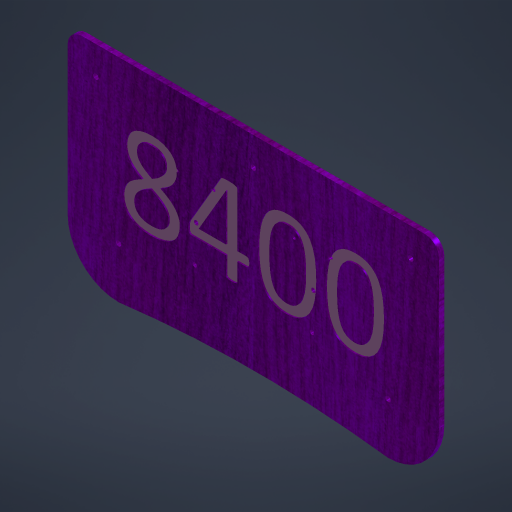
# Autodesk Inventor part: FTC Outside Panels
Saved by Autodesk Inventor 2024.2 (Build 282272000, 272)
## iProperties
Created: 2022-09-22
Part Number: FTC Outside Panels
Material: Wood (Oak)
Document SubType Name: Modeling
Designer: Jason
Density: 0.76 g/cm^3
Appearance: Birch - Natural Polished
Mass: 371.39 g
Surface Area: 1832.51 cm^2
Volume: 488.671 cm^3
Author: Allan
Autodesk Inventor part; units mm, degrees
ref_plane "YZ Plane" through (0, 0, 0) normal (1, 0, 0) x (0, 1, 0)
ref_plane "XZ Plane" through (0, 0, 0) normal (0, 1, 0) x (-1, 0, 0)
ref_plane "XY Plane" through (0, 0, 0) normal (0, 0, 1) x (1, 0, 0)
sketch "Sketch1" plane through (0, 0, 0) normal (0, 0, 1) x (1, 0, 0)
  line L0 (0, 0) -> (333.375, 0)
  line L1 (333.375, 0) -> (333.375, 177.8)
  line L2 (320.675, 190.5) -> (12.7, 190.5)
  line L3 (0, 177.8) -> (0, 0)
  circle A0 centre (45.72, 45.72) radius 45.72
  circle A1 centre (287.655, 45.72) radius 45.72
  line L4 (166.6875, 0) -> (166.6875, 7.62)
  arc A2 (287.655, 0) -> (45.72, 0) centre (166.6875, -956.3695) ccw
  arc A3 (12.7, 190.5) -> (0, 177.8) centre (12.7, 177.8) ccw
  arc A4 (333.375, 177.8) -> (320.675, 190.5) centre (320.675, 177.8) ccw
  circle A5 centre (45.72, 45.72) radius 2.413
  circle A6 centre (287.655, 45.72) radius 2.413
  circle A7 centre (25.4, 165.1) radius 2.413
  circle A8 centre (307.975, 165.1) radius 2.413
  line L5 (25.4, 165.1) -> (307.975, 165.1)
  circle A9 centre (166.6875, 165.1) radius 2.413
  ellipse E0 centre (219.2782, 63.3371) end of major axis (219.2708, 65.3371) minor radius 2
  line L6 (219.2782, 45.72) -> (219.2782, 63.3371)
  ellipse E1 centre (114.0968, 63.3371) end of major axis (114.0894, 65.3371) minor radius 2
  line L7 (114.0968, 45.72) -> (114.0968, 63.3371)
  circle A10 centre (219.3091, 79.3382) radius 4.699
  circle A11 centre (114.1277, 79.3382) radius 4.699
  line L8 (219.2782, 95.3392) -> (219.2782, 63.3371)
  line L9 (114.0968, 95.337) -> (114.0968, 63.3371)
  line L10 (45.72, 45.72) -> (114.0968, 45.72)
  line L11 (287.655, 45.72) -> (219.2782, 45.72)
  ellipse E2 centre (235.2526, 128.7087) end of major axis (235.2552, 127.3562) minor radius 1.3525
  ellipse E3 centre (203.2527, 128.6472) end of major axis (203.2553, 127.2947) minor radius 1.3525
  ellipse E4 centre (219.2782, 95.3392) end of major axis (219.2743, 97.3392) minor radius 2
  ellipse E5 centre (219.2782, 95.3392) end of major axis (219.2743, 97.3392) minor radius 2
  ellipse E6 centre (130.0712, 128.7066) end of major axis (130.0738, 127.354) minor radius 1.3525
  ellipse E7 centre (98.0713, 128.6451) end of major axis (98.0739, 127.2925) minor radius 1.3525
  ellipse E8 centre (114.0968, 95.337) end of major axis (114.0929, 97.337) minor radius 2
  ellipse E9 centre (114.0968, 95.337) end of major axis (114.0929, 97.337) minor radius 2
  point P0 (333.375, 190.5)
  point P1 (0, 190.5)
  point P2 (0, 45.72)
  point P3 (333.375, 45.72)
  dimension "d79" = 91.44
  dimension "d80" = 91.44
  dimension "d77" = 333.375
  dimension "d78" = 190.5
  dimension "d81" = 7.62
  dimension "d82" = 12.7
  dimension "d84" = 4.826
  dimension "d85" = 4.826
  dimension "d86" = 4.826
  dimension "d87" = 25.4
  dimension "d88" = 25.4
  dimension "d90" = 4.826
  dimension "d91" = 25.4
  dimension "d92" = 25.4
  dimension "d94" = 4.826
  dimension "d95" = 17.6171
  dimension "d97" = 17.6171
  dimension "d98" = 9.398
  dimension "d99" = 9.398
  dimension "d103" = 68.3768
  dimension "d104" = 68.3768
  constraints: 24 end point, 14 centre point, 7 point on circle, 6 point on line, 6 vertical, 5 horizontal, 4 tangent, 2 coincident, 2 midpoint, 2 parallel, 1 equal radius, 1 perpendicular, 18 other
  measures "d77" distance of point (0, 190.5) point (333.375, 190.5)
  measures "d78" distance of point (333.375, 190.5) L0.end
  measures "d81" distance of L4.start L4.end
  measures "d82" radius of A3
  measures "d84" diameter of A5
  measures "d85" diameter of A6
  measures "d86" diameter of A7
  measures "d87" distance from line of L2 L5.start
  measures "d88" distance from line of L3 L5.start
  measures "d90" diameter of A8
  measures "d91" distance from line of L1 L5.end
  measures "d92" distance from line of L2 L5.end
  measures "d94" diameter of A9
  measures "d95" distance of L6.start L6.end
  measures "d97" distance of L7.start L7.end
  measures "d98" diameter of A10
  measures "d99" diameter of A11
  measures "d103" distance of L10.start L10.end
  measures "d104" distance of L11.start L11.end
extrude "Extrusion1" add sketch "Sketch1" along normal blind 4.699 contours A0 A2 | L3 A3 L2 A4 L1 A1 A2 A0 | A2 A1 | A10 L8 | L8 A10 | A11 L9 | L9 A11 picked at (30.9641, 18.3065) picked at (302.4109, 18.3065)
sketch "Sketch9" plane through (0, 0, 4.699) normal (0, 0, 1) x (1, 0, 0)
  line L0 (25.0687, 165.288) -> (307.7817, 165.288) construction
  line L1 (307.7817, 165.288) -> (307.7817, 45.2815) construction
  line L2 (307.7817, 45.2815) -> (25.0687, 45.2815) construction
  line L3 (25.0687, 45.2815) -> (25.0687, 165.288) construction
  spline S0 degree 2 poles (100.6714, 86.825) (100.6714, 81.8881) (97.1655, 74.2324) (90.5114, 68.9377) (80.7807, 66.2188) (74.5559, 66.2188) knots 0 0 0 1 2 3 4 4 4
  spline S1 degree 2 poles (74.5559, 66.2188) (68.6889, 66.2188) (59.459, 68.6515) (52.948, 73.5169) (49.5852, 80.5287) (49.5852, 85.0363) knots 0 0 0 1 2 3 4 4 4
  spline S2 degree 2 poles (49.5852, 85.0363) (49.5852, 88.6138) (51.9463, 94.6239) (56.3108, 99.6324) (62.7503, 104.0684) (66.8286, 106.0718) knots 0 0 0 1 2 3 4 4 4
  spline S3 degree 2 poles (66.8286, 106.0718) (63.3227, 107.8605) (57.8849, 111.9388) (54.1644, 116.6611) (52.2325, 122.0273) (52.2325, 125.247) knots 0 0 0 1 2 3 4 4 4
  spline S4 degree 2 poles (52.2325, 125.247) (52.2325, 129.1822) (55.0945, 136.1941) (60.89, 141.3456) (69.8336, 144.3507) (75.8438, 144.3507) knots 0 0 0 1 2 3 4 4 4
  spline S5 degree 2 poles (75.8438, 144.3507) (81.5677, 144.3507) (89.939, 141.5602) (95.3767, 136.838) (97.9525, 130.3986) (97.9525, 126.678) knots 0 0 0 1 2 3 4 4 4
  spline S6 degree 2 poles (97.9525, 126.678) (97.9525, 123.6729) (96.0207, 118.1636) (92.3001, 113.2983) (86.8624, 109.0053) (83.2849, 107.0735) knots 0 0 0 1 2 3 4 4 4
  spline S7 degree 2 poles (83.2849, 107.0735) (87.5063, 105.0701) (94.0173, 100.7056) (98.3818, 95.6972) (100.6714, 90.1163) (100.6714, 86.825) knots 0 0 0 1 2 3 4 4 4
  spline S8 degree 2 poles (90.4398, 85.7518) (90.4398, 88.4707) (88.4365, 92.8352) (84.4297, 96.6988) (78.4196, 100.2763) (74.4128, 102.2081) knots 0 0 0 1 2 3 4 4 4
  spline S9 degree 2 poles (74.4128, 102.2081) (70.7638, 100.3479) (65.1829, 96.6988) (61.6055, 92.8352) (59.8167, 88.5422) (59.8167, 85.9664) knots 0 0 0 1 2 3 4 4 4
  spline S10 degree 2 poles (59.8167, 85.9664) (59.8167, 80.3141) (67.6156, 74.0893) (75.2714, 74.0893) knots 0 0 0 1 2 2 2
  spline S11 degree 2 poles (75.2714, 74.0893) (82.7841, 74.0893) (90.4398, 80.3856) (90.4398, 85.7518) knots 0 0 0 1 2 2 2
  spline S12 degree 2 poles (88.0072, 125.7479) (88.0072, 128.1805) (86.29, 132.1873) (82.9987, 135.0493) (78.2049, 136.4802) (75.0567, 136.4802) knots 0 0 0 1 2 3 4 4 4
  spline S13 degree 2 poles (75.0567, 136.4802) (68.7604, 136.4802) (62.2494, 130.7563) (62.2494, 125.7479) knots 0 0 0 1 2 2 2
  spline S14 degree 2 poles (62.2494, 125.7479) (62.2494, 123.4583) (63.8235, 119.5231) (67.1863, 116.0171) (72.2663, 112.6543) (75.7722, 110.8656) knots 0 0 0 1 2 3 4 4 4
  spline S15 degree 2 poles (75.7722, 110.8656) (81.7108, 113.9422) (88.0072, 121.3118) (88.0072, 125.7479) knots 0 0 0 1 2 2 2
  spline S16 degree 2 poles (162.9908, 88.9) (162.9908, 86.9681) (161.7745, 84.7501) (160.7728, 84.7501) knots 0 0 0 1 2 2 2
  line L4 (160.7728, 84.7501) -> (152.1869, 84.7501)
  line L5 (152.1869, 84.7501) -> (152.1869, 68.7946)
  spline S17 degree 2 poles (152.1869, 68.7946) (152.1869, 68.3653) (151.686, 67.7214) (150.4697, 67.2205) (148.5379, 67.0059) (147.0353, 67.0059) knots 0 0 0 1 2 3 4 4 4
  spline S18 degree 2 poles (147.0353, 67.0059) (145.6043, 67.0059) (143.6725, 67.2205) (142.5277, 67.7214) (142.0984, 68.3653) (142.0984, 68.7946) knots 0 0 0 1 2 3 4 4 4
  line L6 (142.0984, 68.7946) -> (142.0984, 84.7501)
  line L7 (142.0984, 84.7501) -> (111.046, 84.7501)
  spline S19 degree 2 poles (111.046, 84.7501) (110.4021, 84.7501) (109.472, 85.1079) (108.6849, 86.038) (108.3987, 87.8267) (108.3987, 89.1862) knots 0 0 0 1 2 3 4 4 4
  spline S20 degree 2 poles (108.3987, 89.1862) (108.3987, 90.331) (108.5418, 92.0481) (108.828, 93.5507) (109.472, 94.8386) (109.8297, 95.6256) knots 0 0 0 1 2 3 4 4 4
  line L8 (109.8297, 95.6256) -> (136.8753, 141.7749)
  spline S21 degree 2 poles (136.8753, 141.7749) (137.1615, 142.2042) (138.3063, 142.9197) (140.0951, 143.4205) (142.7424, 143.5636) (144.5311, 143.5636) knots 0 0 0 1 2 3 4 4 4
  spline S22 degree 2 poles (144.5311, 143.5636) (146.5345, 143.5636) (149.468, 143.2774) (151.2567, 142.7766) (152.1869, 142.0611) (152.1869, 141.4887) knots 0 0 0 1 2 3 4 4 4
  line L9 (152.1869, 141.4887) -> (152.1869, 93.0498)
  line L10 (152.1869, 93.0498) -> (160.7728, 93.0498)
  spline S23 degree 2 poles (160.7728, 93.0498) (161.7745, 93.0498) (162.9908, 90.9749) (162.9908, 88.9) knots 0 0 0 1 2 2 2
  line L11 (142.0984, 134.6915) -> (141.9553, 134.6915)
  line L12 (141.9553, 134.6915) -> (117.6286, 93.0498)
  line L13 (117.6286, 93.0498) -> (142.0984, 93.0498)
  line L14 (142.0984, 93.0498) -> (142.0984, 134.6915)
  spline S24 degree 2 poles (223.0922, 105.4279) (223.0922, 96.6988) (220.3734, 82.3174) (213.9339, 71.9428) (203.6308, 66.2188) (196.0466, 66.2188) knots 0 0 0 1 2 3 4 4 4
  spline S25 degree 2 poles (196.0466, 66.2188) (188.9632, 66.2188) (179.161, 71.2988) (173.1508, 81.2442) (170.6466, 95.6972) (170.6466, 105.1417) knots 0 0 0 1 2 3 4 4 4
  spline S26 degree 2 poles (170.6466, 105.1417) (170.6466, 113.7991) (173.437, 128.2521) (179.8049, 138.6267) (190.108, 144.3507) (197.6207, 144.3507) knots 0 0 0 1 2 3 4 4 4
  spline S27 degree 2 poles (197.6207, 144.3507) (204.7756, 144.3507) (214.5779, 139.2707) (220.588, 129.3253) (223.0922, 114.8724) (223.0922, 105.4279) knots 0 0 0 1 2 3 4 4 4
  spline S28 degree 2 poles (212.7891, 104.7839) (212.7891, 110.4363) (212.0021, 119.4515) (210.3565, 126.3918) (207.8522, 131.3287) (204.3463, 134.62) (199.8387, 136.051) (197.0483, 136.051) knots 0 0 0 1 2 3 4 5 6 6 6
  spline S29 degree 2 poles (197.0483, 136.051) (192.0398, 136.051) (185.8151, 131.3287) (182.2376, 123.1721) (180.9497, 112.1535) (180.9497, 105.7856) knots 0 0 0 1 2 3 4 4 4
  spline S30 degree 2 poles (180.9497, 105.7856) (180.9497, 97.3428) (182.7384, 85.3941) (186.5305, 77.9529) (192.4691, 74.5186) (196.6905, 74.5186) knots 0 0 0 1 2 3 4 4 4
  spline S31 degree 2 poles (196.6905, 74.5186) (199.9818, 74.5186) (204.9187, 76.5935) (208.4962, 80.5287) (210.8573, 86.038) (212.2883, 92.7636) (212.7891, 100.5625) (212.7891, 104.7839) knots 0 0 0 1 2 3 4 5 6 6 6
  spline S32 degree 2 poles (283.9091, 105.4279) (283.9091, 96.6988) (281.1903, 82.3174) (274.7508, 71.9428) (264.4477, 66.2188) (256.8635, 66.2188) knots 0 0 0 1 2 3 4 4 4
  spline S33 degree 2 poles (256.8635, 66.2188) (249.7801, 66.2188) (239.9779, 71.2988) (233.9677, 81.2442) (231.4635, 95.6972) (231.4635, 105.1417) knots 0 0 0 1 2 3 4 4 4
  spline S34 degree 2 poles (231.4635, 105.1417) (231.4635, 113.7991) (234.2539, 128.2521) (240.6218, 138.6267) (250.9249, 144.3507) (258.4376, 144.3507) knots 0 0 0 1 2 3 4 4 4
  spline S35 degree 2 poles (258.4376, 144.3507) (265.5925, 144.3507) (275.3948, 139.2707) (281.4049, 129.3253) (283.9091, 114.8724) (283.9091, 105.4279) knots 0 0 0 1 2 3 4 4 4
  spline S36 degree 2 poles (273.606, 104.7839) (273.606, 110.4363) (272.819, 119.4515) (271.1734, 126.3918) (268.6691, 131.3287) (265.1632, 134.62) (260.6556, 136.051) (257.8652, 136.051) knots 0 0 0 1 2 3 4 5 6 6 6
  spline S37 degree 2 poles (257.8652, 136.051) (252.8567, 136.051) (246.632, 131.3287) (243.0545, 123.1721) (241.7666, 112.1535) (241.7666, 105.7856) knots 0 0 0 1 2 3 4 4 4
  spline S38 degree 2 poles (241.7666, 105.7856) (241.7666, 97.3428) (243.5553, 85.3941) (247.3474, 77.9529) (253.286, 74.5186) (257.5074, 74.5186) knots 0 0 0 1 2 3 4 4 4
  spline S39 degree 2 poles (257.5074, 74.5186) (260.7987, 74.5186) (265.7356, 76.5935) (269.3131, 80.5287) (271.6742, 86.038) (273.1052, 92.7636) (273.606, 100.5625) (273.606, 104.7839) knots 0 0 0 1 2 3 4 5 6 6 6
  point P0 (0, 0)
  constraints: 2 other
extrude "Extrusion9" cut sketch "Sketch9" against normal blind 1.27
body "Solid1"
